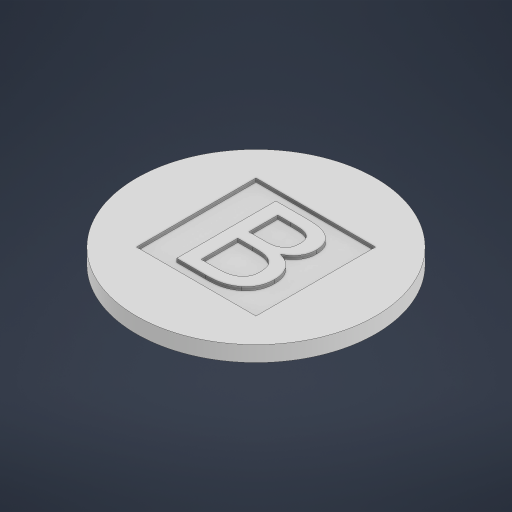
# Autodesk Inventor part: TopMarkerPreset
Saved by Autodesk Inventor 2023.2 (Build 272271030, 271C)
## iProperties
Created: 2023-05-05
Part Number: TopMarkerPreset
Material: Generic
Document SubType Name: Modeling
Designer: Elias Braun
Density: 1 g/cm^3
Appearance: Default
Author: Elias Braun
Autodesk Inventor part; units mm, degrees
ref_plane "YZ Plane" through (0, 0, 0) normal (1, 0, 0) x (0, 1, 0)
ref_plane "XZ Plane" through (0, 0, 0) normal (0, 1, 0) x (-1, 0, 0)
ref_plane "XY Plane" through (0, 0, 0) normal (0, 0, 1) x (1, 0, 0)
sketch "Sketch1" plane through (0, 0, 0) normal (0, 1, 0) x (-1, 0, 0)
  circle A0 centre (0, 0) radius 20
  dimension "d0" = 40
  constraints: 1 centre point, 1 coincident
  measures "d0" diameter of A0
extrude "Extrusion1" add sketch "Sketch1" along normal blind 2.6
sketch "Sketch2" plane through (0, 2.6, 0) normal (0, 1, 0) x (1, 0, 0)
  line L0 (-10, -10) -> (-10, 10)
  line L1 (-10, 10) -> (10, 10)
  line L2 (10, 10) -> (10, -10)
  line L3 (10, -10) -> (-10, -10)
  line L4 (-10, -10) -> (10, 10) construction
  line L5 (-10, 10) -> (10, -10) construction
  point P0 (0, 0)
  dimension "d3" = 20
  dimension "d4" = 20
  constraints: 12 end point, 2 midpoint, 2 parallel, 1 perpendicular, 1 vertical
  measures "d3" distance of L0.start L0.end
  measures "d4" distance of L0.end L1.end
extrude "Extrusion2" cut sketch "Sketch2" against normal blind 0.6
sketch "Sketch3" plane through (0, 2, 0) normal (0, 1, 0) x (1, 0, 0)
  line L0 (-6.6897, 8.3364) -> (6.7624, 8.3364) construction
  line L1 (6.7624, 8.3364) -> (6.7624, -8.2636) construction
  line L2 (6.7624, -8.2636) -> (-6.6897, -8.2636) construction
  line L3 (-6.6897, -8.2636) -> (-6.6897, 8.3364) construction
  spline S0 degree 2 poles (6.2513, -3.1653) (6.2513, -4.4029) (5.3096, -6.2996) (4.5294, -6.9184) knots 0 0 0 1 2 2 2
  spline S1 degree 2 poles (4.5294, -6.9184) (3.5877, -7.6448) (1.4488, -8.2636) (-0.2461, -8.2636) knots 0 0 0 1 2 2 2
  line L4 (-0.2461, -8.2636) -> (-5.0082, -8.2636)
  line L5 (-5.0082, -8.2636) -> (-5.0082, 8.3364)
  line L6 (-5.0082, 8.3364) -> (-0.6094, 8.3364)
  spline S2 degree 2 poles (-0.6094, 8.3364) (1.1663, 8.3364) (2.942, 8.1077) (3.7492, 7.6637) knots 0 0 0 1 2 2 2
  spline S3 degree 2 poles (3.7492, 7.6637) (4.6505, 7.1929) (5.471, 5.6459) (5.471, 4.5966) knots 0 0 0 1 2 2 2
  spline S4 degree 2 poles (5.471, 4.5966) (5.471, 3.4263) (4.2334, 1.5699) (3.1438, 1.0453) knots 0 0 0 1 2 2 2
  line L7 (3.1438, 1.0453) -> (3.1438, 0.9646)
  spline S5 degree 2 poles (3.1438, 0.9646) (4.6235, 0.561) (6.2513, -1.5779) (6.2513, -3.1653) knots 0 0 0 1 2 2 2
  spline S6 degree 2 poles (3.9509, -3.2594) (3.9509, -2.3178) (3.4129, -1.1071) (2.6057, -0.6766) knots 0 0 0 1 2 2 2
  spline S7 degree 2 poles (2.6057, -0.6766) (2.0811, -0.4076) (0.8435, -0.2461) (-0.3, -0.2461) knots 0 0 0 1 2 2 2
  line L8 (-0.3, -0.2461) -> (-2.8021, -0.2461)
  line L9 (-2.8021, -0.2461) -> (-2.8021, -6.3803)
  line L10 (-2.8021, -6.3803) -> (-1.0129, -6.3803)
  spline S8 degree 2 poles (-1.0129, -6.3803) (0.4399, -6.3803) (2.108, -6.1113) (2.7537, -5.6808) knots 0 0 0 1 2 2 2
  spline S9 degree 2 poles (2.7537, -5.6808) (3.3725, -5.2369) (3.9509, -4.1338) (3.9509, -3.2594) knots 0 0 0 1 2 2 2
  spline S10 degree 2 poles (3.1707, 4.2872) (3.1707, 4.8791) (2.7671, 5.767) (2.3232, 6.0226) knots 0 0 0 1 2 2 2
  spline S11 degree 2 poles (2.3232, 6.0226) (1.7851, 6.3185) (0.4803, 6.453) (-0.6901, 6.453) knots 0 0 0 1 2 2 2
  line L11 (-0.6901, 6.453) -> (-2.8021, 6.453)
  line L12 (-2.8021, 6.453) -> (-2.8021, 1.5968)
  line L13 (-2.8021, 1.5968) -> (-0.3, 1.5968)
  spline S12 degree 2 poles (-0.3, 1.5968) (0.7359, 1.5968) (1.7179, 1.812) (2.2425, 2.1483) knots 0 0 0 1 2 2 2
  spline S13 degree 2 poles (2.2425, 2.1483) (2.7537, 2.4712) (3.1707, 3.507) (3.1707, 4.2872) knots 0 0 0 1 2 2 2
  point P0 (0, 0)
  constraints: 2 other
extrude "Extrusion3" add sketch "Sketch3" along normal blind 0.6
body "Solid1"
